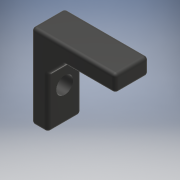
# Autodesk Inventor part: support
Saved by Autodesk Inventor 2018 (Build 220112000, 112)
## iProperties
Created: 2018-05-31
Part Number: support
Material: Plastic, Opaque Black
Document SubType Name: Modeling
Designer: Z. Deniz
Density: 0.952 g/cm^3
Appearance: Smooth - Black
Author: Z. Deniz
Autodesk Inventor part; units mm, degrees
ref_plane "YZ Plane" through (0, 0, 0) normal (1, 0, 0) x (0, 1, 0)
ref_plane "XZ Plane" through (0, 0, 0) normal (0, 1, 0) x (-1, 0, 0)
ref_plane "XY Plane" through (0, 0, 0) normal (0, 0, 1) x (1, 0, 0)
sketch "Sketch2" plane through (0, 0, 0) normal (0, 1, 0) x (-1, 0, 0)
  line L0 (0, 0) -> (0, -20)
  line L1 (0, 0) -> (-20, 0)
  line L2 (0, -20) -> (5, -20)
  line L3 (5, -20) -> (5, 5)
  line L4 (5, 5) -> (-20, 5)
  line L5 (-20, 5) -> (-20, 0)
  dimension "d0" = 20
  dimension "d1" = 20
  dimension "d3" = 5
  dimension "d4" = 25
  dimension "d5" = 90
  dimension "d6" = 25
  constraints: 12 end point, 3 horizontal, 1 perpendicular, 1 vertical
  measures "d0" distance of L0.start L0.end
  measures "d1" distance of L0.start L1.end
  measures "d3" distance of L0.end L2.end
  measures "d4" distance of L2.end L3.end
  measures "d5" angle of L3 L2
  measures "d6" distance of L3.end L4.end
extrude "Extrusion1" add sketch "Sketch2" along normal blind 10
sketch "Sketch3" plane through (0, 0, 0) normal (1, 0, 0) x (0, 0, -1)
  line L0 (20, 0) -> (20, 10) construction
  line L1 (20, 5) -> (0, 5) construction
  circle A0 centre (10, 5) radius 2.5
  point P0 (0, 0)
  dimension "d9" = 5
  dimension "d10" = 10
  constraints: 2 end point, 2 midpoint, 1 centre point, 1 horizontal
  measures "d9" diameter of A0
  measures "d10" distance from line of L0 A0.centre
extrude "Extrusion2" cut sketch "Sketch3" against normal blind 5
chamfer "Chamfer1" distance 5 angle 45 1 edges at (0, 5, 0)
fillet "Fillet1" radius 1 21 edges at (20, 5, 0) (12.5, 0, 0) (20, 0, 2.5) (7.5, 0, 5) (2.5, 0, -2.5) (0, 5, -5) (5, 5, 0) (2.5, 10, -2.5) (12.5, 10, 0) (20, 10, 2.5) (20, 5, 5) (0, 10, -12.5) (0, 5, -20) (-2.5, 10, -20) (-5, 5, -20) (-2.5, 0, -20) (0, 0, -12.5) (-5, 0, -7.5) (-5, 5, 5) (-5, 10, -7.5) (7.5, 10, 5)
body "Solid1"
